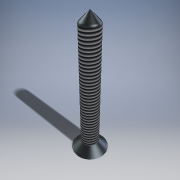
# Autodesk Inventor part: screw
Saved by Autodesk Inventor 2019 (Build 230136000, 136)
## iProperties
Created: 2020-05-25
Part Number: screw
Material: Generic
Document SubType Name: Modeling
Designer: Manoj
Mass: 0.138227 g
Surface Area: 2.37606 cm^2
Volume: 0.138227 cm^3
Density: 1 g/cm^3
Appearance: Iron Gray
Author: Manoj
Autodesk Inventor part; units mm, degrees
ref_plane "YZ Plane" through (0, 0, 0) normal (1, 0, 0) x (0, 1, 0)
ref_plane "XZ Plane" through (0, 0, 0) normal (0, 1, 0) x (-1, 0, 0)
ref_plane "XY Plane" through (0, 0, 0) normal (0, 0, 1) x (1, 0, 0)
sketch "Sketch1" plane through (0, 0, 0) normal (1, 0, 0) x (0, 1, 0)
  line L0 (0, 0) -> (10, 0)
  line L1 (0, 0) -> (-10, 0)
  line L2 (10, 0) -> (8.5858, 1.4142)
  line L3 (8.5858, 1.4142) -> (-10, 1.4142)
  line L4 (-10, 1.4142) -> (-10, 0)
  line L5 (-10, 1.4142) -> (-11.453, 1.4142) construction
  line L6 (-10, 1.4142) -> (-11.4142, 2.8284)
  line L7 (-10, 0) -> (-12.8284, 0)
  line L8 (-11.4142, 2.8284) -> (-11.4142, 0)
  dimension "d0" = 10
  dimension "d1" = 10
  dimension "d2" = 2
  dimension "d3" = 45
  dimension "d4" = 2
  dimension "d8" = 45
  constraints: 18 end point, 4 horizontal, 1 midpoint, 1 perpendicular, 1 point on line
  measures "d0" distance of L0.start L0.end
  measures "d1" distance of L0.start L1.end
  measures "d2" distance of L0.end L2.end
  measures "d3" angle of L0 L2
  measures "d4" distance of L3.end L6.end
  measures "d8" angle of L5 L6
revolve "Revolution1" add sketch "Sketch1" angle 360 about axis through (0, 0, 0) along (0, 1, 0)
fillet "Fillet1" radius 0.5 1 edges at (0, 8.5858, -1.4142)
sketch "Sketch3" plane through (0, -11.4142, 0) normal (0, -1, 0) x (1, 0, 0)
  line L0 (0.2, 1.2) -> (-0.2, 1.2)
  line L1 (-0.2, 1.2) -> (-0.2, -1.2)
  line L2 (-0.2, -1.2) -> (0.2, -1.2)
  line L3 (0.2, -1.2) -> (0.2, 1.2)
  line L4 (1.2, 0.2) -> (-1.2, 0.2)
  line L5 (-1.2, 0.2) -> (-1.2, -0.2)
  line L6 (-1.2, -0.2) -> (1.2, -0.2)
  line L7 (1.2, -0.2) -> (1.2, 0.2)
  point P0 (0, 0)
  dimension "d28" = 0.2
  dimension "d29" = 0.2
  dimension "d30" = 1.2
  dimension "d31" = 1.2
  dimension "d32" = 1.2
  dimension "d33" = 1.2
  dimension "d34" = 0.2
  dimension "d35" = 0.2
  constraints: 16 end point, 4 parallel, 2 horizontal, 2 perpendicular
  measures "d28" distance from line of L3 point (0, 0)
  measures "d29" distance from line of point (0, 0) L1
  measures "d30" distance from line of point (0, 0) L0
  measures "d31" distance from line of L2 point (0, 0)
  measures "d32" distance from line of L7 point (0, 0)
  measures "d33" distance from line of L5 point (0, 0)
  measures "d34" distance from line of point (0, 0) L4
  measures "d35" distance from line of L6 point (0, 0)
extrude "Extrusion1" cut sketch "Sketch3" against normal blind 1.25
thread "Thread2" size "M3x0.5" class "4g6g" standard "ISO Metric profile" full length
body "Solid1"
